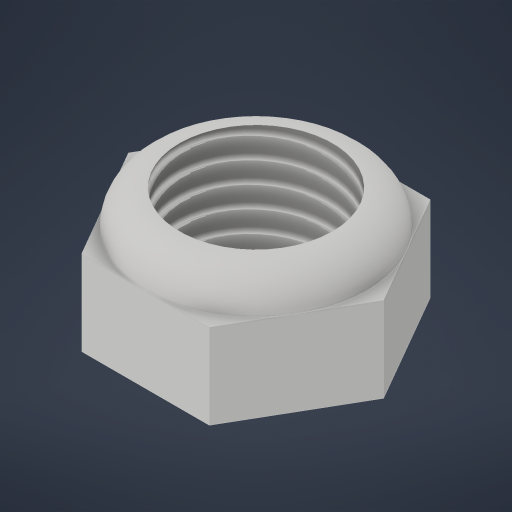
# Autodesk Inventor part: Tuerca
Saved by Autodesk Inventor 2023 (Build 270158000, 158)
## iProperties
Created: 2019-10-31
Part Number: Tuerca
Material: Generic
Document SubType Name: Modeling
Designer: Familia Lopez
Density: 1 g/cm^3
Appearance: Default
Author: Familia Lopez
Autodesk Inventor part; units mm, degrees
ref_plane "YZ Plane" through (0, 0, 0) normal (1, 0, 0) x (0, 1, 0)
ref_plane "XZ Plane" through (0, 0, 0) normal (0, 1, 0) x (-1, 0, 0)
ref_plane "XY Plane" through (0, 0, 0) normal (0, 0, 1) x (1, 0, 0)
sketch "Sketch1" plane through (0, 0, 0) normal (0, 1, 0) x (-1, 0, 0)
  line L0 (0, 0) -> (0, -6.5) construction
  line L1 (-3.7528, -6.5) -> (-7.5056, 0)
  line L2 (-7.5056, 0) -> (-3.7528, 6.5)
  line L3 (-3.7528, 6.5) -> (3.7528, 6.5)
  line L4 (3.7528, 6.5) -> (7.5056, 0)
  line L5 (7.5056, 0) -> (3.7528, -6.5)
  line L6 (3.7528, -6.5) -> (-3.7528, -6.5)
  dimension "d0" = 6.5
  constraints: 14 end point, 1 coincident, 1 midpoint, 1 vertical, 13 other
  measures "d0" distance of L0.start L0.end
extrude "Extrusion1" add sketch "Sketch1" against normal blind 5
sketch "Sketch2" plane through (0, 0, 0) normal (0, 1, 0) x (1, 0, 0)
  circle A0 centre (0, 0) radius 6.5
  constraints: 1 centre point, 1 coincident
extrude "Extrusion2" add sketch "Sketch2" along normal blind 2
fillet "Fillet1" radius 2 1 edges at (-6.5, 2, 0)
sketch "Sketch3" plane through (0, 2, 0) normal (0, 1, 0) x (1, 0, 0)
  circle A0 centre (0, 0) radius 4.5
  constraints: 1 centre point, 1 coincident
extrude "Extrusion3" cut sketch "Sketch3" against normal blind 7
thread "Thread1" size "M9x1.25" class "6H" standard "ANSI Metric M Profile" full length
body "Solid1"
